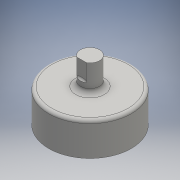
# Autodesk Inventor part: sprag_fill
Saved by Autodesk Inventor 2016 (Build 200138000, 138)
## iProperties
Created: 2017-07-02
Part Number: sprag_fill
Material: Generic
Document SubType Name: Modeling
Designer: ALIREZA
Density: 1 g/cm^3
Appearance: Default
Author: ALIREZA
Autodesk Inventor part; units mm, degrees
ref_plane "YZ Plane" through (0, 0, 0) normal (1, 0, 0) x (0, 1, 0)
ref_plane "XZ Plane" through (0, 0, 0) normal (0, 1, 0) x (-1, 0, 0)
ref_plane "XY Plane" through (0, 0, 0) normal (0, 0, 1) x (1, 0, 0)
sketch "Sketch1" plane through (0, 0, 0) normal (0, 0, 1) x (1, 0, 0)
  circle A0 centre (0, 0) radius 11.5
  dimension "d0" = 23
  constraints: 1 centre point, 1 coincident
  measures "d0" diameter of A0
sketch "Sketch2" plane through (0, 0, 0) normal (0, 0, 1) x (1, 0, 0)
  circle A0 centre (0, 0) radius 13
  dimension "d1" = 26
  constraints: 1 centre point, 1 coincident
  measures "d1" diameter of A0
extrude "Extrusion1" add sketch "Sketch2" along normal blind 10.5
extrude "Extrusion2" cut sketch "Sketch1" along normal blind 9
fillet "Fillet1" radius 0.5 1 edges at (-11.5, 0, 9)
sketch "Sketch3" plane through (0, 0, 10.5) normal (0, 0, 1) x (1, 0, 0)
  circle A0 centre (0, 0) radius 3
  dimension "d7" = 6
  constraints: 1 centre point, 1 coincident
  measures "d7" diameter of A0
extrude "Extrusion3" add sketch "Sketch3" along normal blind 8.5
fillet "Fillet2" radius 1 1 edges at (-13, 0, 10.5)
fillet "Fillet3" radius 1.5 1 edges at (-3, 0, 10.5)
sketch "Sketch4" plane through (0, 0, 19) normal (0, 0, 1) x (1, 0, 0)
  arc A0 (-1.5, -2.5981) -> (1.5154, -2.5891) centre (0, 0) ccw
  line L0 (-1.5, -2.5981) -> (1.5154, -2.5891)
  circle A1 centre (0, 0) radius 3 projected
  constraints: 2 end point, 2 point on circle, 1 centre point, 2 other
extrude "Extrusion4" cut sketch "Sketch4" against normal blind 5.5 contours L0 A0
sketch "Sketch5" plane through (0, 0, 10.5) normal (0, 0, 1) x (1, 0, 0)
  point P0 (0, 0)
sketch "Sketch8" plane through (0, 0, 0) normal (0, 0, -1) x (-1, 0, 0)
  circle A0 centre (0, 0) radius 11.5 projected
  line L0 (0.0233, -10.9901) -> (-0.4767, -10.9901)
  line L1 (-0.4767, -10.9901) -> (-0.4767, -11.4901)
  line L2 (0.0233, -10.9901) -> (0.5233, -10.9901)
  line L3 (0.5233, -10.9901) -> (0.5233, -11.4881)
  dimension "d27" = 0.5
  dimension "d28" = 0.5
  dimension "d32" = 0.5
  constraints: 8 end point, 2 perpendicular, 2 point on circle, 1 horizontal
  measures "d27" distance of L0.start L0.end
  measures "d28" distance of L0.start L2.end
  measures "d32" distance of L0.end L1.end
extrude "Extrusion7" add sketch "Sketch8" against normal up to next contours L1 L0 L2 L3 A0 picked at (-0.1989, -11.1598)
fillet "Fillet4" radius 1 1 edges at (0.0077, -2.5936, 13.5)
body "Solid1"
